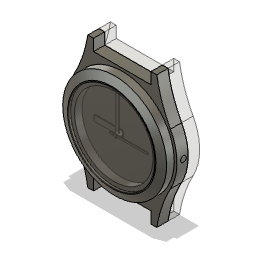
watch-model1 (Autodesk Fusion 360 design; units mm, degrees)
Autodesk Fusion 360 part; units mm, degrees
sketch "Sketch1" plane through (0, 0, 0) normal (0, 0, 1) x (1, 0, 0) in component "besel"
  circle A0 centre (0, 0) radius 18.05
  circle A1 centre (0, 0) radius 14.65
  dimension "d1" = 36.1
  dimension "d2" = 29.3
  constraint coincident A0.centre A1.centre
  constraint concentric A0 A1
  measures "d1" diameter of A0
  measures "d2" diameter of A1
extrude "Extrude1" add sketch "Sketch1" along normal blind 0.35 contours A0 picked at (16.7949, -1.6246) makes body 1 in component "besel"
sketch "Sketch2" plane through (0, 0, 0.35) normal (0, 0, 1) x (1, 0, 0) in component "besel"
  circle A0 centre (0, 0) radius 14.65
  circle A1 centre (0, 0) radius 18.05
  circle A2 centre (0, 0) radius 13.65
  dimension "d5" = 27.3
  constraint concentric A0 A2
  measures "d5" diameter of A2
extrude "Extrude2" add sketch "Sketch2" along normal blind 3.3 contours A0 | A1 picked at (14.2113, -1.406) picked at (16.7949, -1.6246) bodies 1 in component "besel"
sketch "Sketch3" plane through (0, 0, 3.65) normal (0, 0, 1) x (1, 0, 0) in component "besel"
  circle A0 centre (0, 0) radius 13.65
  circle A1 centre (0, 0) radius 18.05
  circle A2 centre (0, 0) radius 15
  dimension "d8" = 30
  constraint coincident A0.centre A1.centre
  measures "d8" diameter of A2
extrude "Extrude3" cut sketch "Sketch3" against normal blind 0.7 contours A2 picked at (14.4942, -0.7452) bodies 1 in component "besel"
sketch "Sketch4" plane through (0, 0, 0) normal (0, 0, -1) x (-1, 0, 0) in component "besel"
  circle A0 centre (0, 0) radius 14.65
  circle A1 centre (0, 0) radius 18.05
  circle A2 centre (0, 0) radius 16.5
  dimension "d11" = 33
  constraint concentric A0 A2
  measures "d11" diameter of A2
extrude "Extrude4" add sketch "Sketch4" along normal blind 1.05 contours A2 picked at (15.8219, -0.8197) bodies 1 in component "besel"
chamfer "Chamfer1" distance 2.7 distance2 1 1 edges at (-16.8285, -6.5272, 3.65) measured on face at (16.9103, -1.6419, 3.65) on bodies 1 in component "besel"
sketch "Sketch1 (2)" plane through (0, 0, 0) normal (0, 0, -1) x (-1, 0, 0) in component "top-frame"
  circle A0 centre (0, 0) radius 16.5
  circle A1 centre (0, 0) radius 18.05
  line L0 (27.5, -27.5) -> (-27.5, -27.5)
  line L1 (-27.5, -27.5) -> (-27.5, 27.5)
  line L2 (-27.5, 27.5) -> (27.5, 27.5)
  line L3 (27.5, 27.5) -> (27.5, -27.5)
  line L4 (27.5, -27.5) -> (-27.5, 27.5) construction
  line L5 (-27.5, -27.5) -> (27.5, 27.5) construction
  dimension "d16" = 55
  dimension "d17" = 55
  constraint horizontal L0
  constraint perpendicular L0 L1
  constraint parallel L0 L2
  constraint parallel L1 L3
  constraint coincident L4 A0.centre
  constraint coincident L5 A0.centre
  constraint coincident A0.centre A1.centre
  measures "d16" distance of L1.end L2.end
  measures "d17" distance of L0.end L1.end
extrude "Extrude1'" add sketch "Sketch1 (2)" along normal blind 3.9 separate body contours A1 | L0 L1 L2 L3 picked at (17.4661, -0.8967) picked at (-0.4496, -24.3332) makes body 2 in component "top-frame"
sketch "Sketch1 (3)" plane through (0, 0, -3.9) normal (0, 0, -1) x (-1, 0, 0)
  circle A0 centre (0, 0) radius 16.5
  line L0 (27.5, 27.5) -> (-27.5, 27.5)
  line L1 (-27.5, 27.5) -> (-27.5, -27.5)
  line L2 (-27.5, -27.5) -> (27.5, -27.5)
  line L3 (27.5, -27.5) -> (27.5, 27.5)
  circle A1 centre (0, 0) radius 14.7
  dimension "d20" = 29.4
  constraint coincident A0.centre A1.centre
  measures "d20" diameter of A1
extrude "Extrude2'" add sketch "Sketch1 (3)" against normal blind 2.8 contours A0 picked at (15.7838, -1.55) bodies 2 in component "top-frame"
sketch "Sketch1 (4)" plane through (0, 0, 0.35) normal (0, 0, -1) x (-1, 0, 0) in component "dial"
  circle A0 centre (0, 0) radius 13.65
  circle A1 centre (0, 0) radius 14.65
  circle A2 centre (0, 0) radius 0.8
  dimension "d23" = 1.6
  constraint concentric A0 A2
  measures "d23" diameter of A2
extrude "Extrude1''" add sketch "Sketch1 (4)" along normal blind 0.6 separate body contours A0 | A1 picked at (9.3129, -0.7179) picked at (14.2113, -1.406) makes body 3 in component "dial"
sketch "Sketch1 (5)" plane through (0, 0, -0.25) normal (0, 0, -1) x (-1, 0, 0) in component "movement"
  circle A0 centre (0, 0) radius 0.8
  circle A1 centre (0, 0) radius 14.65
  circle A2 centre (0, 0) radius 14.7
  dimension "d26" = 29.4
  constraint coincident A0.centre A1.centre
  measures "d26" diameter of A2
extrude "Extrude1'''" add sketch "Sketch1 (5)" along normal blind 6 separate body contours A0 | A1 A2 picked at (0.273, 0.1637) picked at (9.9788, 0.7278) makes body 4 in component "movement"
sketch "Sketch2 (2)" plane through (0, 0, -6.25) normal (0, 0, -1) x (-1, 0, 0) in component "movement"
  circle A0 centre (0, 0) radius 14.65
  circle A1 centre (0, 0) radius 13.9
  dimension "d29" = 27.8
  constraint concentric A0 A1
  measures "d29" diameter of A1
extrude "Extrude2''" cut sketch "Sketch2 (2)" against normal blind 3 contours A0 picked at (14.2937, -1.4184) bodies 4 in component "movement"
sketch "Sketch4 (2)" plane through (0, 0, 0) normal (1, 0, 0) x (0, 0, -1) in component "movement"
  line L0 (0.2615, 0) -> (2.2615, 0) construction
  line L1 (2.2615, 0) -> (2.2615, -1) construction
  line L2 (2.2615, -1) -> (0.2615, -1) construction
  line L3 (0.2615, -1) -> (0.2615, 0) construction
  circle A0 centre (2.2615, 0) radius 1
  dimension "d32" = 2
  dimension "d33" = 1
  dimension "d34" = 2
  constraint horizontal L0
  constraint vertical L1
  constraint horizontal L2
  constraint vertical L3
  constraint coincident L0.end L1.start
  measures "d32" distance of L0.start L0.end
  measures "d33" distance of L0.start L2.end
  measures "d34" diameter of A0
extrude "Extrude3'" add sketch "Sketch4 (2)" along normal blind 20 separate body contours A0 picked at (2.2431, 0.441) makes body 5 in component "movement"
extrude "Extrude4'" add sketch "Sketch1 (5)" against normal blind 2.7 contours A0 picked at (0.273, 0.1637) bodies 4 in component "movement"
sketch "Sketch5" plane through (0, 0, 2.45) normal (0, 0, 1) x (1, 0, 0) in component "movement"
  circle A0 centre (0, 0) radius 0.8
  line L0 (-1.9526, 0.3166) -> (11.17, 0.3166)
  line L1 (11.17, 0.3166) -> (11.17, -0.3166)
  line L2 (11.17, -0.3166) -> (-1.9526, -0.3166)
  line L3 (-1.9526, -0.3166) -> (-1.9526, 0.3166)
  constraint horizontal L0
  constraint vertical L1
  constraint horizontal L2
  constraint vertical L3
extrude "Extrude5" add sketch "Sketch5" against normal blind 0.2 separate body contours A0 L0 L2 | A0 L0 L1 L2 | A0 L0 L2 L3 picked at (0.2231, 0) picked at (7.7133, 0) picked at (-1.5684, 0) makes body 6 in component "movement"
sketch "Sketch6" plane through (0, 0, 2.45) normal (0, 0, 1) x (1, 0, 0) in component "movement"
  circle A0 centre (0, 0) radius 0.8
  circle A1 centre (0, 0) radius 0.5
  constraint coincident A0.centre A1.centre
extrude "Extrude6" add sketch "Sketch6" along normal blind 0.2 contours A1 picked at (0.2632, -0.1794) bodies 4 6 in component "movement"
sketch "Sketch1 (6)" plane through (0, 0, 2.95) normal (0, 0, 1) x (1, 0, 0) in component "cristal"
  circle A0 centre (0, 0) radius 13.65
  circle A1 centre (0, 0) radius 15
  circle A2 centre (0, 0) radius 15
  constraint coincident A0.centre A1.centre
extrude "Extrude1''''" add sketch "Sketch1 (6)" along normal blind 1 separate body contours A0 | A1 A2 picked at (-3.4867, 5.1141) picked at (14.4942, -0.7452) makes body 7 in component "cristal"
ref_plane "WorkPlane1" through (0, 0, 0.85) normal (0, 0, 1) x (1, 0, 0) in component "movement"
sketch "Sketch7" plane through (0, 0, 0.85) normal (0, 0, 1) x (1, 0, 0) in component "movement"
  line L0 (1, 1) -> (-9, 1)
  line L1 (-9, 1) -> (-9, -1)
  line L2 (-9, -1) -> (1, -1)
  line L3 (1, -1) -> (1, 1)
  constraint horizontal L0
  constraint vertical L1
  constraint horizontal L2
  constraint vertical L3
extrude "Extrude7" add sketch "Sketch7" against normal blind 0.2 separate body contours L0 L1 L2 L3 picked at (-5.6667, 0.3333) makes body 8 in component "movement"
ref_plane "WorkPlane2" through (0, 0, 1.75) normal (0, 0, -1) x (-1, 0, 0) in component "movement"
sketch "Sketch8" plane through (0, 0, 1.75) normal (0, 0, -1) x (-1, 0, 0) in component "movement"
  line L0 (-0.5, -1) -> (0.5, -1)
  line L1 (0.5, -1) -> (0.5, 12.5)
  line L2 (0.5, 12.5) -> (-0.5, 12.5)
  line L3 (-0.5, 12.5) -> (-0.5, -1)
  constraint horizontal L0
  constraint vertical L1
  constraint horizontal L2
  constraint vertical L3
extrude "Extrude8" add sketch "Sketch8" along normal blind 0.2 separate body contours L0 L1 L2 L3 picked at (-0.1667, 8) makes body 9 in component "movement"
sketch "Sketch1 (7)" plane through (0, 0, -3.9) normal (0, 0, -1) x (-1, 0, 0) in component "bottom-frame"
  circle A0 centre (0, 0) radius 14.7
  line L0 (27.5, 27.5) -> (-27.5, 27.5)
  line L1 (-27.5, 27.5) -> (-27.5, -27.5)
  line L2 (-27.5, -27.5) -> (27.5, -27.5)
  line L3 (27.5, -27.5) -> (27.5, 27.5)
  circle A1 centre (0, 0) radius 14
  line L4 (27.5, -27.5) -> (-27.5, -27.5)
  line L5 (-27.5, -27.5) -> (-27.5, 27.5)
  line L6 (-27.5, 27.5) -> (27.5, 27.5)
  line L7 (27.5, 27.5) -> (27.5, -27.5)
  line L8 (27.5, -27.5) -> (-27.5, 27.5) construction
  line L9 (-27.5, -27.5) -> (27.5, 27.5) construction
  dimension "d51" = 55
  dimension "d52" = 55
  constraint concentric A0 A1
  constraint horizontal L4
  constraint perpendicular L4 L5
  constraint parallel L4 L6
  constraint parallel L5 L7
  constraint coincident L8 A0.centre
  constraint coincident L9 A0.centre
  constraint coincident A0.centre A1.centre
  measures "d51" distance of L0.end L0.start
  measures "d52" distance of L1.end L0.end
extrude "Extrude1'''''" add sketch "Sketch1 (7)" along normal blind 4 separate body contours A0 | L0 L1 L2 L3 L4 L5 L6 L7 picked at (14.4119, -0.7303) picked at (-0.3662, -23.2196) makes body 10 in component "bottom-frame"
sketch "Sketch2 (3)" plane through (0, 0, -7.9) normal (0, 0, -1) x (-1, 0, 0)
  circle A0 centre (0, 0) radius 14
  line L0 (27.5, 27.5) -> (-27.5, 27.5)
  line L1 (-27.5, 27.5) -> (-27.5, -27.5)
  line L2 (-27.5, -27.5) -> (27.5, -27.5)
  line L3 (27.5, -27.5) -> (27.5, 27.5)
extrude "Extrude2'''" add sketch "Sketch2 (3)" against normal blind 1 contours A0 picked at (4.8081, -3.2781) bodies 10 in component "bottom-frame"
sketch "Sketch3 (2)" plane through (0, 0, 0) normal (0, 0, 1) x (1, 0, 0)
  circle A0 centre (0, 0) radius 16.5
  line L0 (27.5, 27.5) -> (-27.5, 27.5)
  line L1 (-27.5, 27.5) -> (-27.5, -27.5)
  line L2 (-27.5, -27.5) -> (27.5, -27.5)
  line L3 (27.5, -27.5) -> (27.5, 27.5)
  line L4 (-10, 30) -> (10, 30) construction
  line L5 (10, 30) -> (10, -29) construction
  line L6 (10, -29) -> (-10, -29) construction
  line L7 (-10, -29) -> (-10, 30) construction
  line L8 (-10, 30) -> (-12, 30) construction
  line L9 (-12, 30) -> (-12, -29) construction
  line L10 (-12, -29) -> (-10, -29) construction
  line L11 (-10, -29) -> (-10, 30) construction
  line L12 (10, 30) -> (12, 30) construction
  line L13 (12, 30) -> (12, -29) construction
  line L14 (12, -29) -> (10, -29) construction
  line L15 (10, -29) -> (10, 30) construction
  line L16 (-10, 19) -> (10, 19)
  line L17 (10, 19) -> (10, 23)
  line L18 (-10, 23) -> (-10, 19)
  line L19 (-10, -19) -> (10, -19)
  line L20 (10, -19) -> (10, -23)
  line L21 (-10, -23) -> (-10, -19)
  line L22 (-12, 23) -> (-10, 23)
  line L23 (10, 23) -> (12, 23)
  line L24 (-12, -23) -> (-10, -23)
  line L25 (10, -23) -> (12, -23)
  circle A1 centre (0, 0) radius 19
  line L26 (-20, 9) -> (19, 9) construction
  arc A2 (-16.7332, 9) -> (-12, 23) centre (-55.7792, 30.001) ccw
  arc A3 (12, 23) -> (16.7332, 9) centre (55.7792, 30.001) ccw
  line L27 (10, -19) -> (-19.8159, -19) construction
  line L28 (-19.8159, -19) -> (-19.8159, -9) construction
  line L29 (-19.8159, -9) -> (10, -9) construction
  line L30 (10, -9) -> (10, -19) construction
  line L31 (10, -9) -> (25, -9) construction
  arc A4 (-12, -23) -> (-16.7332, -9) centre (-55.7792, -30.001) ccw
  arc A5 (16.7332, -9) -> (12, -23) centre (55.7792, -30.001) ccw
  dimension "d57" = 10
  constraint horizontal L4
  constraint vertical L5
  constraint horizontal L6
  constraint vertical L7
  constraint horizontal L8
  constraint vertical L9
  constraint horizontal L10
  constraint vertical L11
  constraint horizontal L12
  constraint vertical L13
  constraint horizontal L14
  constraint vertical L15
  constraint horizontal L16
  constraint vertical L17
  constraint vertical L18
  constraint coincident L5 L17.end
  constraint coincident L7 L16.start
  constraint horizontal L19
  constraint vertical L20
  constraint vertical L21
  constraint coincident L15 L20.end
  constraint coincident L7 L19.start
  constraint coincident L9 L24.start
  constraint coincident L13 L25.end
  constraint perpendicular L13 L24
  constraint coincident L9 L22.start
  constraint coincident L13 L23.end
  constraint perpendicular L13 L22
  constraint collinear L22 L23
  constraint collinear L24 L25
  constraint coincident A0.centre A1.centre
  constraint perpendicular L13 L26
  constraint tangent A1 A2
  constraint coincident A1 A2.start
  constraint coincident L26 A2.start
  constraint tangent A1 A3
  constraint coincident L26 A3.end
  constraint coincident A1 A3.end
  constraint horizontal L27
  constraint vertical L28
  constraint horizontal L29
  constraint vertical L30
  constraint perpendicular L3 L31
  constraint tangent A1 A4
  constraint coincident A1 A4.end
  constraint coincident L29 A4.end
  constraint tangent A1 A5
  constraint coincident L31 A5.start
  constraint coincident A1 A5.start
  measures "d57" distance of L19.end L29.end
extrude "Extrude3''" cut sketch "Sketch3 (2)" against normal blind 40 contours L0 L1 L2 L3 picked at (-24.6509, 0.4461) bodies 2 in component "top-frame"
extrude "Extrude9" cut sketch "Sketch3 (2)" against normal blind 40 contours L0 L1 L2 L3 picked at (-24.6509, 0.4461) bodies 5 in component "movement"
extrude "Extrude3'''" cut sketch "Sketch3 (2)" against normal blind 40 contours L0 L1 L2 L3 picked at (-24.6509, 0.4461) bodies 10 in component "bottom-frame"
component "besel" placed x (1, 0, 0) y (0, 1, 0) z (0, 0, 1) at (0, 0, 0)
component "top-frame" placed x (1, 0, 0) y (0, 1, 0) z (0, 0, 1) at (0, 0, 0)
component "dial" placed x (1, 0, 0) y (0, 1, 0) z (0, 0, 1) at (0, 0, 0)
component "movement" placed x (1, 0, 0) y (0, 1, 0) z (0, 0, 1) at (0, 0, 0)
component "cristal" placed x (1, 0, 0) y (0, 1, 0) z (0, 0, 1) at (0, 0, 0)
component "bottom-frame" placed x (1, 0, 0) y (0, 1, 0) z (0, 0, 1) at (0, 0, 0)
equation "d3 = 1.4 mm - 1.05 mm"
